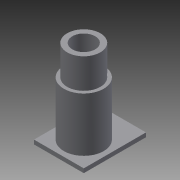
# Autodesk Inventor part: Tube_Part
Saved by Autodesk Inventor 2014 (Build 180170000, 170)
## iProperties
Created: 2014-05-02
Part Number: Tube_Part
Material: Generic
Document SubType Name: Modeling
Designer: Alex
Density: 1 g/cm^3
Appearance: Default
Author: Alex
Autodesk Inventor part; units mm, degrees
ref_plane "YZ Plane" through (0, 0, 0) normal (1, 0, 0) x (0, 1, 0)
ref_plane "XZ Plane" through (0, 0, 0) normal (0, 1, 0) x (-1, 0, 0)
ref_plane "XY Plane" through (0, 0, 0) normal (0, 0, 1) x (1, 0, 0)
sketch "Sketch1" plane through (0, 0, 0) normal (0, 1, 0) x (-1, 0, 0)
  circle A0 centre (0, 0) radius 6.096
  circle A1 centre (0, 0) radius 3.4925
  dimension "d0" = 12.192
  dimension "d1" = 6.985
  constraints: 2 centre point, 2 coincident
  measures "d0" diameter of A0
  measures "d1" diameter of A1
extrude "Extrusion1" add sketch "Sketch1" along normal blind 15.24
sketch "Sketch2" plane through (0, 15.24, 0) normal (0, 1, 0) x (1, 0, 0)
  circle A0 centre (0, 0) radius 3.4925 projected
  circle A1 centre (0, 0) radius 6.096 projected
  circle A2 centre (0, 0) radius 3.4925
  circle A3 centre (0, 0) radius 5.08
  dimension "d4" = 10.16
  constraints: 2 centre point, 2 coincident, 1 concentric
  measures "d4" diameter of A3
extrude "Extrusion2" add sketch "Sketch2" along normal blind 9.144 contours A3
sketch "Sketch3" plane through (0, 0, 0) normal (0, -1, 0) x (1, 0, 0)
  circle A0 centre (0, 0) radius 3.4925 projected
  circle A1 centre (0, 0) radius 6.096 projected
  circle A2 centre (0, 0) radius 3.4925
  circle A3 centre (0, 0) radius 6.096
  constraints: 2 centre point, 2 coincident, 2 concentric
extrude "Extrusion3" add sketch "Sketch3" along normal blind 2.54
sketch "Sketch4" plane through (0, -2.54, 0) normal (0, -1, 0) x (1, 0, 0)
  circle A0 centre (0, 0) radius 6.096 projected
  circle A1 centre (0, 0) radius 6.096
  line L0 (-7.62, 7.62) -> (7.62, 7.62)
  line L1 (7.62, 7.62) -> (7.62, -11.43)
  line L2 (7.62, -11.43) -> (-7.62, -11.43)
  line L3 (-7.62, -11.43) -> (-7.62, 7.62)
  dimension "d12" = 15.24
  dimension "d13" = 19.05
  dimension "d14" = 7.62
  dimension "d15" = 7.62
  constraints: 8 end point, 2 parallel, 1 centre point, 1 coincident, 1 concentric, 1 horizontal, 1 perpendicular
  measures "d12" distance between parallel lines of L1 L3
  measures "d13" distance between parallel lines of L2 L0
  measures "d14" distance from line of A0.centre L0
  measures "d15" distance from line of L1 A0.centre
extrude "Extrusion4" add sketch "Sketch4" against normal blind 1.27
body "Solid1"
